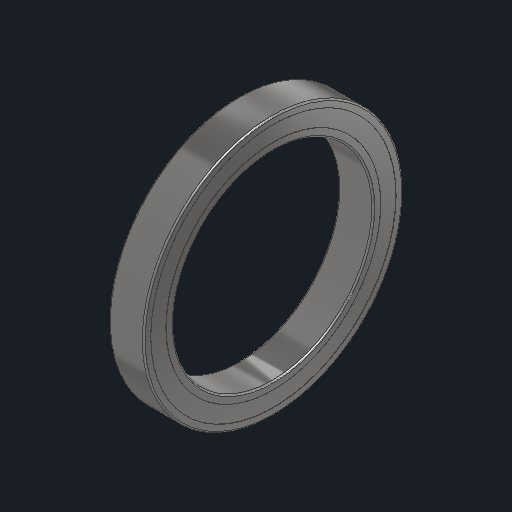
# Autodesk Inventor part: B6808ZZ
Saved by Autodesk Inventor 2022 (Build 260153000, 153)
## iProperties
Category: PARTsolutions
Company: MISUMI
Part Number: B6808ZZ
Material: 鋼、炭素鋼
Catalog Web Link: www.cadenas.de
Description: ミスミ？
Vendor: MISUMI
Document SubType Name: Modeling
Designer: partserver
Manufacturer: MISUMI
Mass: 46.9929 g
Surface Area: 37.2954 cm^2
Volume: 5.98636 cm^3
Density: 7.85 g/cm^3
Appearance: 半つや出し
PSOL_IDENT_0: {$CADENAS_DATA\23d-libs\misumi\metric\12_bearing_holders\sb6010zz.prj},172 {VTYP=3D},{NB=B6808ZZ},{L
PSOL_IDENT_1: INA=B6808ZZ},{NN=B6_ _ _ZZ, SB6_ _ _ZZ},{DATE=22.10.2019 07:39:52},{GEOMDATE=22.10.2019 06:26:04},{V
PSOL_IDENT_2: ERSION=},{LINEID=370},{WBVAR=TS},{WBNUMERIC=}  {NB=B6808ZZ},{LINA=B6808ZZ},{KT=DUMMY},{PN=B6808ZZ},{
PSOL_IDENT_3: TS=},{TS1= '', 'Steel', 'S', 'Stainless Steel'},{MAT=52100 Bearing Steel},{BN=6808ZZ},{DD=40},{D=52}
PSOL_IDENT_4: ,{B=7},{RR=0.3},{CR=5.10},{COR=4.40},{CRS=5.10},{CRSS=4.18},{CORS=4.40},{CORSS=3.34},{DD1=1.00},{R1=
PSOL_IDENT_5: 1.00},{R2=1.0},{DSMIN=42.0},{DSMAX=43.00},{DS1=43.00},{DDHH=50.0},{R=0.3},{MASS=33},{MASS11=33},{AA=
PSOL_IDENT_6: 6.8390},{BB=1.4100},{CC=1.5000},{TYS=w/o Retaining Ring}
NB: B6808ZZ
NN: B6_ _ _ZZ, SB6_ _ _ZZ
NT: Deep Groove Ball Bearings - Double Shield Type
NBSYN: $PN.
LINA: B6808ZZ
CATALOG: Misumi
PN: B6808ZZ
TS: Steel
MAT: 52100 Bearing Steel
BN: 6808ZZ
DD: 40
D: 52
B: 7
RR: 0.3
CR: 5.10
COR: 4.40
DSMIN: 42
DSMAX: 43
DDHH: 50
R: 0.3
MASS: 33
SUPPLIER: MISUMI
ARTICLENO: B6808ZZ
BOMINFO: B6808ZZ
CREATOR: CADENAS GmbH
購入先: ミスミ
在庫数: 2.0
代替品型番: C-B6808ZZ
Title: B6808ZZ
Author: Cadenas PARTsolutions
Comments: Deep Groove Ball Bearings - Double Shield Type
Autodesk Inventor part; units mm, degrees
sketch "Sketch_1" plane through (0, 0, 0) normal (0, 0, 1) x (1, 0, 0)
  line L0 (7, 0) -> (0, 0)
  arc A0 (0, 20.3) -> (0.3, 20) centre (0.3, 20.3) ccw
  line L1 (0.3, 20) -> (6.7, 20)
  arc A1 (6.7, 20) -> (7, 20.3) centre (6.7, 20.3) ccw
  line L2 (7, 20.3) -> (7, 21.5)
  line L3 (7, 21.5) -> (6.9195, 21.5)
  line L4 (6.9195, 21.5) -> (6.9195, 24.59)
  line L5 (6.9195, 24.59) -> (7, 24.59)
  line L6 (7, 24.59) -> (7, 25.7)
  arc A2 (7, 25.7) -> (6.7, 26) centre (6.7, 25.7) ccw
  line L7 (6.7, 26) -> (0.3, 26)
  arc A3 (0.3, 26) -> (0, 25.7) centre (0.3, 25.7) ccw
  line L8 (0, 25.7) -> (0, 24.59)
  line L9 (0, 24.59) -> (0.0805, 24.59)
  line L10 (0.0805, 24.59) -> (0.0805, 21.5)
  line L11 (0.0805, 21.5) -> (0, 21.5)
  line L12 (0, 21.5) -> (0, 20.3)
  constraints: 26 end point, 8 point on circle, 4 centre point
revolve "Revolution1" add sketch "Sketch_1" angle 360 about axis through (7, 0, 0) along (1, 0, 0)
ref_plane "center_point_XY" through (3.5, 0, 0) normal (1, 0, 0) x (0, 0, -1)
ref_plane "center_point_YZ" through (3.5, 0, 0) normal (0, 0, -1) x (0, 1, 0)
ref_plane "center_point_ZX" through (3.5, 0, 0) normal (0, 1, 0) x (1, 0, 0)
ref_plane "to_housing_XY" through (0, 0, 0) normal (1, 0, 0) x (0, 0, -1)
ref_plane "to_housing_YZ" through (0, 0, 0) normal (0, 0, -1) x (0, 1, 0)
ref_plane "to_housing_ZX" through (0, 0, 0) normal (0, 1, 0) x (1, 0, 0)
ref_plane "to_ring_XY" through (6.839, 0, 0) normal (1, 0, 0) x (0, 0, -1)
ref_plane "to_ring_YZ" through (6.839, 0, 0) normal (0, 0, -1) x (0, 1, 0)
ref_plane "to_ring_ZX" through (6.839, 0, 0) normal (0, 1, 0) x (1, 0, 0)
body "Solid1"
